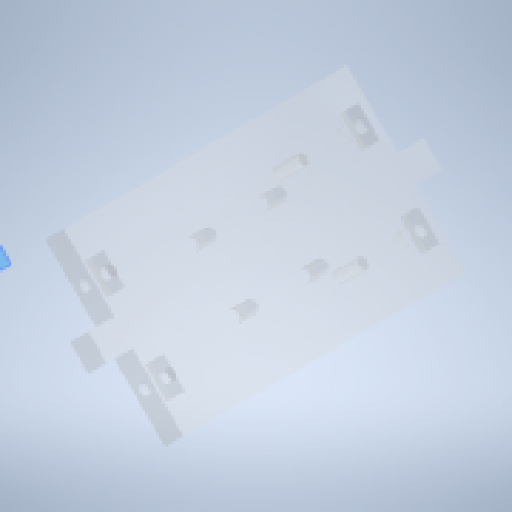
# Autodesk Inventor part: foot_2
Saved by Autodesk Inventor 2024 (Build 280153000, 153)
## iProperties
Created: 2024-09-05
Part Number: foot_2
Material: PMMA 플라스틱
Document SubType Name: Modeling
Designer: Eungang
Density: 1.188 g/cm^3
Appearance: 폴리카보네이트 - 선명
Mass: 18.11 g
Surface Area: 72.1845 cm^2
Volume: 15.2441 cm^3
Author: Eungang
Autodesk Inventor part; units mm, degrees
ref_plane "YZ Plane" through (0, 0, 0) normal (1, 0, 0) x (0, 1, 0)
ref_plane "XZ Plane" through (0, 0, 0) normal (0, 1, 0) x (-1, 0, 0)
ref_plane "XY Plane" through (0, 0, 0) normal (0, 0, 1) x (1, 0, 0)
sketch "스케치1" plane through (0, 0, 0) normal (0, 0, 1) x (1, 0, 0)
  arc A0 (25.8359, 13.6528) -> (21.7064, 16.0915) centre (22.8544, 13.3199) ccw projected
  line L0 (21.1279, 15.8519) -> (21.7064, 16.0915) projected
  arc A1 (21.1279, 15.8519) -> (19.2893, 12.7982) centre (22.276, 13.0803) ccw projected
  arc A2 (12.7982, 19.2893) -> (19.2893, 12.7982) centre (12.1212, 12.1212) ccw projected
  arc A3 (12.7982, 19.2893) -> (15.8519, 21.1279) centre (13.0803, 22.276) ccw projected
  line L1 (16.0915, 21.7064) -> (15.8519, 21.1279) projected
  arc A4 (16.0915, 21.7064) -> (13.6528, 25.8359) centre (13.3199, 22.8544) ccw projected
  arc A5 (13.6528, 25.8359) -> (2.3631, 21.8792) centre (12.1212, 12.1212) ccw projected
  line L2 (-25.9212, -6.405) -> (2.3631, 21.8792) projected
  line L3 (-18.2844, -14.0418) -> (-25.9212, -6.405) projected
  line L4 (-14.0418, -9.7991) -> (-18.2844, -14.0418) projected
  line L5 (-9.7991, -14.0418) -> (-14.0418, -9.7991) projected
  line L6 (-14.0418, -18.2844) -> (-9.7991, -14.0418) projected
  line L7 (-6.405, -25.9212) -> (-14.0418, -18.2844) projected
  line L8 (21.8792, 2.3631) -> (-6.405, -25.9212) projected
  arc A6 (21.8792, 2.3631) -> (25.8359, 13.6528) centre (12.1212, 12.1212) ccw projected
  circle A7 centre (23.1212, 12.1212) radius 1.2812 projected
  circle A8 centre (19.8993, 4.343) radius 1.2812 projected
  circle A9 centre (1.1212, 12.1212) radius 1.2812 projected
  circle A10 centre (12.1212, 1.1212) radius 1.2812 projected
  circle A11 centre (4.343, 4.343) radius 1.2812 projected
  circle A12 centre (4.343, 19.8993) radius 1.2812 projected
  circle A13 centre (12.1212, 23.1212) radius 1.2812 projected
  circle A14 centre (-7.1121, -20.9714) radius 1.25 projected
  circle A15 centre (-20.9714, -7.1121) radius 1.25 projected
  line L9 (-25.9212, -6.405) -> (-18.2844, -14.0418)
  line L10 (-14.0418, -9.7991) -> (-18.2844, -14.0418)
  line L11 (-14.0418, -9.7991) -> (-9.7991, -14.0418)
  line L12 (-14.0418, -18.2844) -> (-9.7991, -14.0418)
  line L13 (-21.6785, -2.1624) -> (-14.0418, -9.7991)
  line L14 (-21.6785, -2.1624) -> (-25.9212, -6.405)
  line L15 (-9.7991, -14.0418) -> (-2.1624, -21.6785)
  line L16 (-2.1624, -21.6785) -> (-6.405, -25.9212)
  line L17 (-6.405, -25.9212) -> (-14.0418, -18.2844)
  line L18 (-18.2844, -14.0418) -> (-14.0418, -18.2844)
  point P0 (0, 0)
  constraints: 20 end point, 6 collinear, 4 point on line, 2 perpendicular
extrude "돌출1" add sketch "스케치1" along normal blind 50.4 contours L8 L7 L6 L15 | L6 L18 L4 L5 | L4 L3 L2 L13 | A14 | A15
sketch "스케치2" plane through (0, 0, 0) normal (0, 0, -1) x (-1, 0, 0)
  line L0 (2.1624, -21.6785) -> (21.6785, -2.1624) projected
  arc A0 (-21.7064, 16.0915) -> (-25.8359, 13.6528) centre (-22.8544, 13.3199) ccw projected
  arc A1 (-25.8359, 13.6528) -> (-21.8792, 2.3631) centre (-12.1212, 12.1212) ccw projected
  line L1 (-21.8792, 2.3631) -> (6.405, -25.9212) projected
  line L2 (6.405, -25.9212) -> (14.0418, -18.2844) projected
  line L3 (14.0418, -18.2844) -> (9.7991, -14.0418) projected
  line L4 (9.7991, -14.0418) -> (14.0418, -9.7991) projected
  line L5 (14.0418, -9.7991) -> (18.2844, -14.0418) projected
  line L6 (18.2844, -14.0418) -> (25.9212, -6.405) projected
  line L7 (25.9212, -6.405) -> (-2.3631, 21.8792) projected
  arc A2 (-2.3631, 21.8792) -> (-13.6528, 25.8359) centre (-12.1212, 12.1212) ccw projected
  arc A3 (-13.6528, 25.8359) -> (-16.0915, 21.7064) centre (-13.3199, 22.8544) ccw projected
  line L8 (-16.0915, 21.7064) -> (-15.8519, 21.1279) projected
  arc A4 (-15.8519, 21.1279) -> (-12.7982, 19.2893) centre (-13.0803, 22.276) ccw projected
  arc A5 (-19.2893, 12.7982) -> (-12.7982, 19.2893) centre (-12.1212, 12.1212) ccw projected
  arc A6 (-19.2893, 12.7982) -> (-21.1279, 15.8519) centre (-22.276, 13.0803) ccw projected
  line L9 (-21.1279, 15.8519) -> (-21.7064, 16.0915) projected
  circle A7 centre (-23.1212, 12.1212) radius 1.2812 projected
  circle A8 centre (-19.8993, 4.343) radius 1.2812 projected
  circle A9 centre (-1.1212, 12.1212) radius 1.2812 projected
  circle A10 centre (-12.1212, 1.1212) radius 1.2812 projected
  circle A11 centre (-4.343, 4.343) radius 1.2812 projected
  circle A12 centre (-4.343, 19.8993) radius 1.2812 projected
  circle A13 centre (-12.1212, 23.1212) radius 1.2812 projected
  circle A14 centre (7.1121, -20.9714) radius 1.25 projected
  circle A15 centre (20.9714, -7.1121) radius 1.25 projected
  line L10 (25.9212, -6.405) -> (6.405, -25.9212) projected
  point P0 (0, 0)
extrude "돌출2" add sketch "스케치2" along normal blind 6 contours L0 L5 L10 L3
sketch "스케치3" plane through (0, 0, 50.4) normal (0, 0, 1) x (1, 0, 0)
  arc A0 (25.8359, 13.6528) -> (21.7064, 16.0915) centre (22.8544, 13.3199) ccw projected
  line L0 (21.1279, 15.8519) -> (21.7064, 16.0915) projected
  arc A1 (21.1279, 15.8519) -> (19.2893, 12.7982) centre (22.276, 13.0803) ccw projected
  arc A2 (12.7982, 19.2893) -> (19.2893, 12.7982) centre (12.1212, 12.1212) ccw projected
  arc A3 (12.7982, 19.2893) -> (15.8519, 21.1279) centre (13.0803, 22.276) ccw projected
  line L1 (16.0915, 21.7064) -> (15.8519, 21.1279) projected
  arc A4 (16.0915, 21.7064) -> (13.6528, 25.8359) centre (13.3199, 22.8544) ccw projected
  arc A5 (13.6528, 25.8359) -> (2.3631, 21.8792) centre (12.1212, 12.1212) ccw projected
  line L2 (-25.9212, -6.405) -> (2.3631, 21.8792) projected
  line L3 (-18.2844, -14.0418) -> (-25.9212, -6.405) projected
  line L4 (-14.0418, -9.7991) -> (-18.2844, -14.0418) projected
  line L5 (-9.7991, -14.0418) -> (-14.0418, -9.7991) projected
  line L6 (-14.0418, -18.2844) -> (-9.7991, -14.0418) projected
  line L7 (-6.405, -25.9212) -> (-14.0418, -18.2844) projected
  line L8 (21.8792, 2.3631) -> (-6.405, -25.9212) projected
  arc A6 (21.8792, 2.3631) -> (25.8359, 13.6528) centre (12.1212, 12.1212) ccw projected
  circle A7 centre (23.1212, 12.1212) radius 1.2812 projected
  circle A8 centre (19.8993, 4.343) radius 1.2812 projected
  circle A9 centre (1.1212, 12.1212) radius 1.2812 projected
  circle A10 centre (12.1212, 1.1212) radius 1.2812 projected
  circle A11 centre (4.343, 4.343) radius 1.2812 projected
  circle A12 centre (4.343, 19.8993) radius 1.2812 projected
  circle A13 centre (12.1212, 23.1212) radius 1.2812 projected
  circle A14 centre (-7.1121, -20.9714) radius 1.25 projected
  circle A15 centre (-20.9714, -7.1121) radius 1.25 projected
  line L9 (-25.9212, -6.405) -> (-6.405, -25.9212) projected
  point P0 (0, 0)
extrude "돌출3" add sketch "스케치3" along normal blind 6 contours L9 L4 L5 L6
sketch "스케치4" plane through (0, 0, 0) normal (0, 0, -1) x (-1, 0, 0)
  arc A0 (-21.7064, 16.0915) -> (-25.8359, 13.6528) centre (-22.8544, 13.3199) ccw projected
  arc A1 (-25.8359, 13.6528) -> (-21.8792, 2.3631) centre (-12.1212, 12.1212) ccw projected
  line L0 (-21.8792, 2.3631) -> (6.405, -25.9212) projected
  line L1 (6.405, -25.9212) -> (14.0418, -18.2844) projected
  line L2 (14.0418, -18.2844) -> (9.7991, -14.0418) projected
  line L3 (9.7991, -14.0418) -> (14.0418, -9.7991) projected
  line L4 (14.0418, -9.7991) -> (18.2844, -14.0418) projected
  line L5 (18.2844, -14.0418) -> (25.9212, -6.405) projected
  line L6 (25.9212, -6.405) -> (-2.3631, 21.8792) projected
  arc A2 (-2.3631, 21.8792) -> (-13.6528, 25.8359) centre (-12.1212, 12.1212) ccw projected
  arc A3 (-13.6528, 25.8359) -> (-16.0915, 21.7064) centre (-13.3199, 22.8544) ccw projected
  line L7 (-16.0915, 21.7064) -> (-15.8519, 21.1279) projected
  arc A4 (-15.8519, 21.1279) -> (-12.7982, 19.2893) centre (-13.0803, 22.276) ccw projected
  arc A5 (-19.2893, 12.7982) -> (-12.7982, 19.2893) centre (-12.1212, 12.1212) ccw projected
  arc A6 (-19.2893, 12.7982) -> (-21.1279, 15.8519) centre (-22.276, 13.0803) ccw projected
  line L8 (-21.1279, 15.8519) -> (-21.7064, 16.0915) projected
  circle A7 centre (-23.1212, 12.1212) radius 1.2812 projected
  circle A8 centre (-19.8993, 4.343) radius 1.2812 projected
  circle A9 centre (-1.1212, 12.1212) radius 1.2812 projected
  circle A10 centre (-12.1212, 1.1212) radius 1.2812 projected
  circle A11 centre (-4.343, 4.343) radius 1.2812 projected
  circle A12 centre (-4.343, 19.8993) radius 1.2812 projected
  circle A13 centre (-12.1212, 23.1212) radius 1.2812 projected
  circle A14 centre (7.1121, -20.9714) radius 1.25 projected
  circle A15 centre (20.9714, -7.1121) radius 1.25 projected
  point P0 (0, 0)
extrude "돌출4" cut sketch "스케치4" against normal blind 6 contours A14 | A15
sketch "스케치5" plane through (0, 0, 50.4) normal (0, 0, 1) x (1, 0, 0)
  arc A0 (25.8359, 13.6528) -> (21.7064, 16.0915) centre (22.8544, 13.3199) ccw projected
  line L0 (21.1279, 15.8519) -> (21.7064, 16.0915) projected
  arc A1 (21.1279, 15.8519) -> (19.2893, 12.7982) centre (22.276, 13.0803) ccw projected
  arc A2 (12.7982, 19.2893) -> (19.2893, 12.7982) centre (12.1212, 12.1212) ccw projected
  arc A3 (12.7982, 19.2893) -> (15.8519, 21.1279) centre (13.0803, 22.276) ccw projected
  line L1 (16.0915, 21.7064) -> (15.8519, 21.1279) projected
  arc A4 (16.0915, 21.7064) -> (13.6528, 25.8359) centre (13.3199, 22.8544) ccw projected
  arc A5 (13.6528, 25.8359) -> (2.3631, 21.8792) centre (12.1212, 12.1212) ccw projected
  line L2 (-25.9212, -6.405) -> (2.3631, 21.8792) projected
  line L3 (-18.2844, -14.0418) -> (-25.9212, -6.405) projected
  line L4 (-14.0418, -9.7991) -> (-18.2844, -14.0418) projected
  line L5 (-9.7991, -14.0418) -> (-14.0418, -9.7991) projected
  line L6 (-14.0418, -18.2844) -> (-9.7991, -14.0418) projected
  line L7 (-6.405, -25.9212) -> (-14.0418, -18.2844) projected
  line L8 (21.8792, 2.3631) -> (-6.405, -25.9212) projected
  arc A6 (21.8792, 2.3631) -> (25.8359, 13.6528) centre (12.1212, 12.1212) ccw projected
  circle A7 centre (23.1212, 12.1212) radius 1.2812 projected
  circle A8 centre (19.8993, 4.343) radius 1.2812 projected
  circle A9 centre (1.1212, 12.1212) radius 1.2812 projected
  circle A10 centre (12.1212, 1.1212) radius 1.2812 projected
  circle A11 centre (4.343, 4.343) radius 1.2812 projected
  circle A12 centre (4.343, 19.8993) radius 1.2812 projected
  circle A13 centre (12.1212, 23.1212) radius 1.2812 projected
  circle A14 centre (-7.1121, -20.9714) radius 1.25 projected
  circle A15 centre (-20.9714, -7.1121) radius 1.25 projected
  point P0 (0, 0)
extrude "돌출5" cut sketch "스케치5" against normal blind 6 contours A14 | A15
sketch "스케치16" plane through (-21.6785, -2.1624, 0) normal (0.7071068, 0.7071068, 0) x (-0.7071068, 0.7071068, 0)
  line L0 (-27.4, -20.9) -> (-27.4, -14.9) projected
  line L1 (-27.4, -14.9) -> (-17.8, -14.9) projected
  line L2 (-17.8, -14.9) -> (-17.8, -20.9) projected
  line L3 (-27.4, -20.9) -> (-17.8, -20.9) projected
  line L4 (0, 0) -> (0, 50.4) projected
  line L5 (-27.4, -14.9) -> (0, -14.9)
  line L6 (0, -14.9) -> (0, 0)
  line L7 (0, 0) -> (-27.4, 0)
  line L8 (-27.4, 0) -> (-27.4, -14.9)
  line L9 (-0.2, -14.9) -> (-0.2, -20.9) projected
  line L10 (-9.8, -20.9) -> (-0.2, -20.9) projected
  line L11 (-9.8, -20.9) -> (-9.8, -14.9) projected
  line L12 (-9.8, -14.9) -> (-0.2, -14.9) projected
  line L13 (-16.9, -20.9) -> (-16.9, -14.9) projected
  line L14 (-10.7, -20.9) -> (-10.7, -14.9) projected
  line L15 (-16.9, -14.9) -> (-10.7, -14.9)
  line L16 (-10.7, -14.9) -> (-10.7, -20.9)
  line L17 (-10.7, -20.9) -> (-16.9, -20.9)
  line L18 (-16.9, -20.9) -> (-16.9, -14.9)
  line L19 (-16.9, -14.9) -> (-16.8, -14.9)
  line L20 (-10.7, -14.9) -> (-10.8, -14.9)
  line L21 (-10.8, -14.9) -> (-10.8, -21)
  line L22 (-16.8, -14.9) -> (-16.8, -20.9)
  point P0 (-13.8, 0)
  point P1 (-16.8, -14.9)
  point P2 (-10.8, -20.9)
  dimension "d25" = 0.1
  dimension "d26" = 0.1
  constraints: 24 end point, 4 parallel, 4 perpendicular, 3 point on line, 2 horizontal
  measures "d25" distance of L13.end L19.end
  measures "d26" distance of L15.end L20.end
extrude "돌출11" add sketch "스케치16" against normal blind 6 contours L8 L7 L6 L5 L1 | L5 L21 L17 L22
sketch "스케치17" plane through (-14.0418, -9.7991, -14.9) normal (0, 0, -1) x (-0.7071068, -0.7071068, 0)
  line L0 (6, 10.6) -> (-34, 10.6) projected
  arc A0 (-34, 10.6) -> (-45.0739, 4.8949) centre (-34, -3) ccw projected
  arc A1 (-45.0739, 4.8949) -> (-43.6082, 2.05) centre (-43.6082, 3.85) ccw projected
  line L1 (-43.6082, 2.05) -> (-34, 2.05) projected
  arc A2 (-34, -8.05) -> (-34, 2.05) centre (-34, -3) ccw projected
  line L2 (-34, -8.05) -> (-43.6082, -8.05) projected
  arc A3 (-43.6082, -8.05) -> (-45.0739, -10.8949) centre (-43.6082, -9.85) ccw projected
  arc A4 (-45.0739, -10.8949) -> (-34, -16.6) centre (-34, -3) ccw projected
  line L3 (-34, -16.6) -> (6, -16.6) projected
  line L4 (6, -16.6) -> (6, -7) projected
  arc A5 (5.005, -6.1) -> (6, -7) centre (6, -6) ccw projected
  line L5 (5.005, -6.1) -> (0.995, -6.1) projected
  arc A6 (-0.1, -5.005) -> (0.995, -6.1) centre (0, -6) ccw projected
  line L6 (-0.1, -5.005) -> (-0.1, -0.995) projected
  arc A7 (0.995, 0.1) -> (-0.1, -0.995) centre (0, 0) ccw projected
  line L7 (0.995, 0.1) -> (5.005, 0.1) projected
  arc A8 (6, 1) -> (5.005, 0.1) centre (6, 0) ccw projected
  line L8 (6, 1) -> (6, 10.6) projected
  circle A9 centre (-34, -14) radius 1.2812 projected
  circle A10 centre (-41.7782, -10.7782) radius 1.2812 projected
  circle A11 centre (-23, -3) radius 1.2812 projected
  circle A12 centre (-26.2218, 4.7782) radius 1.2812 projected
  circle A13 centre (-26.2218, -10.7782) radius 1.2812 projected
  circle A14 centre (-34, 8) radius 1.2812 projected
  circle A15 centre (-41.7782, 4.7782) radius 1.2812 projected
  circle A16 centre (3, 6.8) radius 1.35
  circle A17 centre (3, -12.8) radius 1.35
  point P0 (-16.8581, -3)
  constraints: 2 centre point
extrude "돌출12" cut sketch "스케치17" against normal blind 6 contours A16 | A17
sketch "스케치18" plane through (0, 0, 50.4) normal (0, 0, 1) x (1, 0, 0)
  line L0 (2.5045, 21.7378) -> (-25.7798, -6.5464) projected
  line L1 (-18.9915, -13.3347) -> (-25.7798, -6.5464) projected
  arc A0 (-17.6516, -13.2675) -> (-18.9915, -13.3347) centre (-18.2844, -14.0418) ccw projected
  line L2 (-17.6516, -13.2675) -> (-14.8161, -10.432) projected
  arc A1 (-13.2675, -10.432) -> (-14.8161, -10.432) centre (-14.0418, -9.7991) ccw projected
  line L3 (-13.2675, -10.432) -> (-10.432, -13.2675) projected
  arc A2 (-10.432, -14.8161) -> (-10.432, -13.2675) centre (-9.7991, -14.0418) ccw projected
  line L4 (-10.432, -14.8161) -> (-13.2675, -17.6516) projected
  arc A3 (-13.3347, -18.9915) -> (-13.2675, -17.6516) centre (-14.0418, -18.2844) ccw projected
  line L5 (-6.5464, -25.7798) -> (-13.3347, -18.9915) projected
  line L6 (-6.5464, -25.7798) -> (21.7378, 2.5045) projected
  arc A4 (21.7378, 2.5045) -> (25.5341, 14.369) centre (12.1212, 12.1212) ccw projected
  arc A5 (25.5341, 14.369) -> (22.4861, 15.3443) centre (23.7589, 14.0715) ccw projected
  line L7 (22.4861, 15.3443) -> (15.6921, 8.5503) projected
  arc A6 (8.5503, 15.6921) -> (15.6921, 8.5503) centre (12.1212, 12.1212) ccw projected
  line L8 (8.5503, 15.6921) -> (15.3443, 22.4861) projected
  arc A7 (15.3443, 22.4861) -> (14.369, 25.5341) centre (14.0715, 23.7589) ccw projected
  arc A8 (14.369, 25.5341) -> (2.5045, 21.7378) centre (12.1212, 12.1212) ccw projected
  circle A9 centre (-7.1121, -20.9714) radius 1.25 projected
  circle A10 centre (12.1212, 23.1212) radius 1.2812 projected
  circle A11 centre (4.343, 19.8993) radius 1.2812 projected
  circle A12 centre (12.1212, 1.1212) radius 1.2812 projected
  circle A13 centre (1.1212, 12.1212) radius 1.2812 projected
  circle A14 centre (4.343, 4.343) radius 1.2812 projected
  circle A15 centre (23.1212, 12.1212) radius 1.2812 projected
  circle A16 centre (19.8993, 4.343) radius 1.2812 projected
  circle A17 centre (-20.9714, -7.1121) radius 1.25 projected
  circle A18 centre (-20.9714, -7.1121) radius 1.25 projected
  line L9 (-18.2844, -14.0418) -> (-14.0418, -9.7991) projected
  line L10 (-14.0418, -9.7991) -> (-21.6785, -2.1624) projected
  line L11 (-21.6785, -2.1624) -> (-25.9212, -6.405) projected
  line L12 (-25.9212, -6.405) -> (-18.2844, -14.0418) projected
  circle A19 centre (-7.1121, -20.9714) radius 1.25 projected
  line L13 (-9.7991, -14.0418) -> (-14.0418, -18.2844) projected
  line L14 (-14.0418, -18.2844) -> (-6.405, -25.9212) projected
  line L15 (-6.405, -25.9212) -> (-2.1624, -21.6785) projected
  line L16 (-2.1624, -21.6785) -> (-9.7991, -14.0418) projected
  point P0 (0, 0)
  point P1 (-21.5371, -2.3038)
  point P2 (-2.3038, -21.5371)
extrude "돌출13" cut sketch "스케치18" against normal through all contours L0 L12 L11 L10 | L16 L15 L14 L6
sketch "스케치20" plane through (-14.0418, -9.7991, 50.4) normal (0.7071068, 0.7071068, 0) x (-0.7071068, 0.7071068, 0)
  line L0 (10.6, -65.3) -> (10.6, 0) projected
  line L1 (0, 0) -> (10.6, 0) projected
  line L2 (0, 0) -> (0, 6) projected
  line L3 (-6, 6) -> (0, 6) projected
  line L4 (-6, 0) -> (-6, 6) projected
  line L5 (-16.6, 0) -> (-6, 0) projected
  line L6 (-16.6, 0) -> (-16.6, -65.3) projected
  line L7 (-16.6, -65.3) -> (-6, -65.3) projected
  line L8 (-6, -65.3) -> (-6, -71.3) projected
  line L9 (-6, -71.3) -> (0, -71.3) projected
  line L10 (0, -71.3) -> (0, -65.3) projected
  line L11 (0, -65.3) -> (10.6, -65.3) projected
  line L12 (-16.6, 0) -> (-16.6, -65.3) projected
  line L13 (-16.6, -32.65) -> (10.6, -32.65)
  line L14 (-3, 6) -> (-3, -71.3)
  line L15 (-3, -32.65) -> (-3, 0)
  line L16 (-5.005, 0) -> (-0.995, 0) projected
  line L17 (-3, 0) -> (-3, -32.65)
  line L18 (-6, -65.3) -> (0, -65.3)
  line L19 (-3, -65.3) -> (-3, -32.65)
  line L20 (-3, -48.975) -> (-16.6, -48.975)
  line L21 (-16.6, -65.3) -> (-16.6, 0) projected
  line L22 (-3, -48.975) -> (-3, -32.65)
  line L23 (-3, -40.8125) -> (-16.6, -40.8125)
  circle A0 centre (-9.8, -40.8125) radius 1.35
  circle A1 centre (3.8, -40.8125) radius 1.35
  circle A2 centre (-9.8, -24.4875) radius 1.35
  circle A3 centre (3.8, -24.4875) radius 1.35
  point P0 (-3, -50.4)
  dimension "d33" = 2.7
  constraints: 18 end point, 9 midpoint, 4 centre point, 4 perpendicular, 3 point on line, 3 symmetric about line, 2 collinear, 3 other
  measures "d33" diameter of A0
extrude "돌출14" cut sketch "스케치20" against normal up to next contours A0 L23 | L23 A0 | A1 | A2 | A3
sketch "스케치21" plane through (-14.0418, -9.7991, 50.4) normal (0.7071068, 0.7071068, 0) x (-0.7071068, 0.7071068, 0)
  circle A0 centre (3.8, -24.4875) radius 1.35 projected
  circle A1 centre (-9.8, -24.4875) radius 1.35 projected
  circle A2 centre (3.8, -40.8125) radius 1.35 projected
  circle A3 centre (-9.8, -40.8125) radius 1.35 projected
  line L0 (10.6, -65.3) -> (10.6, 0) projected
  line L1 (0, 0) -> (10.6, 0) projected
  line L2 (0, 0) -> (0, 6) projected
  line L3 (-6, 6) -> (0, 6) projected
  line L4 (-6, 0) -> (-6, 6) projected
  line L5 (-16.6, 0) -> (-6, 0) projected
  line L6 (-16.6, 0) -> (-16.6, -65.3) projected
  line L7 (-16.6, -65.3) -> (-6, -65.3) projected
  line L8 (-6, -65.3) -> (-6, -71.3) projected
  line L9 (-6, -71.3) -> (0, -71.3) projected
  line L10 (0, -71.3) -> (0, -65.3) projected
  line L11 (0, -65.3) -> (10.6, -65.3) projected
  line L12 (-11.55, 0) -> (-11.55, 6)
  line L13 (-11.55, 0) -> (-11.55, 6)
  line L14 (-14.05, 0) -> (-14.05, 6)
  line L15 (-14.05, -6) -> (-11.55, -6) projected
  line L16 (-11.55, 0) -> (-14.05, 0)
  line L17 (-14.05, 0) -> (-14.05, -6)
  line L18 (-14.05, -6) -> (-11.55, -6)
  line L19 (-11.55, -6) -> (-11.55, 0)
  line L20 (-12.8, -6) -> (-12.8, 0)
  line L21 (-12.8, -3) -> (-9.3, -3)
  line L22 (-12.8, -3) -> (-16.3, -3)
  line L23 (-9.3, -3) -> (-9.3, -4.5)
  line L24 (-9.3, -3) -> (-9.3, -1.5)
  line L25 (-16.3, -3) -> (-16.3, -4.5)
  line L26 (-16.3, -3) -> (-16.3, -1.5)
  line L27 (-9.3, -1.5) -> (-16.3, -1.5)
  line L28 (-16.3, -1.5) -> (-16.3, -4.5)
  line L29 (-16.3, -4.5) -> (-9.3, -4.5)
  line L30 (-9.3, -4.5) -> (-9.3, -1.5)
  line L31 (-3, 6) -> (-3, 1)
  line L32 (6.8, -3) -> (3.3, -3)
  line L33 (6.8, -3) -> (10.3, -3)
  line L34 (3.3, -3) -> (3.3, -4.5)
  line L35 (3.3, -3) -> (3.3, -1.5)
  line L36 (10.3, -3) -> (10.3, -4.5)
  line L37 (10.3, -3) -> (10.3, -1.5)
  line L38 (3.3, -1.5) -> (10.3, -1.5)
  line L39 (10.3, -1.5) -> (10.3, -4.5)
  line L40 (10.3, -4.5) -> (3.3, -4.5)
  line L41 (3.3, -4.5) -> (3.3, -1.5)
  line L42 (10.6, -32.65) -> (-16.6, -32.65)
  line L43 (-14.05, -59.3) -> (-11.55, -59.3)
  line L44 (-14.05, -59.3) -> (-11.55, -59.3)
  line L45 (-12.8, -62.3) -> (-9.3, -62.3)
  line L46 (-12.8, -62.3) -> (-16.3, -62.3)
  line L47 (-9.3, -62.3) -> (-9.3, -60.8)
  line L48 (-9.3, -62.3) -> (-9.3, -63.8)
  line L49 (-16.3, -62.3) -> (-16.3, -60.8)
  line L50 (-16.3, -62.3) -> (-16.3, -63.8)
  line L51 (-9.3, -63.8) -> (-16.3, -63.8)
  line L52 (-16.3, -63.8) -> (-16.3, -60.8)
  line L53 (-16.3, -60.8) -> (-9.3, -60.8)
  line L54 (-9.3, -60.8) -> (-9.3, -63.8)
  line L55 (10.3, -60.8) -> (3.3, -60.8)
  line L56 (10.3, -62.3) -> (10.3, -60.8)
  line L57 (3.3, -62.3) -> (3.3, -60.8)
  line L58 (6.8, -62.3) -> (3.3, -62.3)
  line L59 (6.8, -62.3) -> (10.3, -62.3)
  line L60 (3.3, -62.3) -> (3.3, -63.8)
  line L61 (3.3, -60.8) -> (3.3, -63.8)
  line L62 (3.3, -63.8) -> (10.3, -63.8)
  line L63 (10.3, -62.3) -> (10.3, -63.8)
  line L64 (10.3, -63.8) -> (10.3, -60.8)
  line L65 (10.6, 0) -> (16.6, 0)
  line L66 (16.6, 0) -> (16.6, -65.3)
  line L67 (16.6, -65.3) -> (10.6, -65.3)
  line L68 (10.6, -65.3) -> (10.6, 0)
  line L69 (-16.6, 0) -> (-22.6, 0)
  line L70 (-22.6, 0) -> (-22.6, -65.3)
  line L71 (-22.6, -65.3) -> (-16.6, -65.3)
  line L72 (-16.6, -65.3) -> (-16.6, 0)
  point P0 (-3, -50.4)
  point P1 (-16.3, -1.5)
  point P2 (-9.3, -4.5)
  point P3 (3.3, -4.5)
  point P4 (10.3, -1.5)
  point P5 (-12.8, -59.3)
  dimension "d36" = 3.5
  dimension "d37" = 3.5
  dimension "d38" = 1.5
  dimension "d39" = 1.5
  dimension "d40" = 1.5
  dimension "d43" = 6
  dimension "d44" = 6
  constraints: 120 end point, 31 symmetric about line, 8 parallel, 8 vertical, 6 midpoint, 5 perpendicular, 5 point on line, 4 horizontal, 4 other
  measures "d36" distance of L21.start L21.end
  measures "d37" distance of L21.start L22.end
  measures "d38" distance of L21.end L23.end
  measures "d39" distance of L21.end L24.end
  measures "d40" distance of L22.end L25.end
  measures "d43" distance of L66.end L67.end
  measures "d44" distance of L71.end L70.end
extrude "돌출15" cut sketch "스케치21" against normal up to next contours L27 L20 L22 L17 | L17 L22 L26 L27 | L27 L19 L21 L20 | L22 L20 L29 L17 | L17 L29 L25 L22 | L27 L24 L21 L19 | L21 L19 L29 L20 | L21 L23 L29 L19 | L33 L36 L40 L34 L32 | L32 L35 L38 L37 L33
sketch "스케치22" plane through (-14.0418, -9.7991, 50.4) normal (0.7071068, 0.7071068, 0) x (-0.7071068, 0.7071068, 0)
  line L0 (-9.3, -4.5) -> (-16.3, -4.5) projected
  line L1 (-16.3, -4.5) -> (-16.3, -1.5) projected
  line L2 (-16.3, -1.5) -> (-9.3, -1.5) projected
  line L3 (-9.3, -1.5) -> (-9.3, -4.5) projected
  line L4 (3.3, -1.5) -> (10.3, -1.5) projected
  line L5 (10.3, -1.5) -> (10.3, -4.5) projected
  line L6 (10.3, -4.5) -> (3.3, -4.5) projected
  line L7 (3.3, -4.5) -> (3.3, -1.5) projected
  circle A0 centre (3.8, -24.4875) radius 1.35 projected
  circle A1 centre (-9.8, -24.4875) radius 1.35 projected
  circle A2 centre (3.8, -40.8125) radius 1.35 projected
  circle A3 centre (-9.8, -40.8125) radius 1.35 projected
  line L8 (10.6, -65.3) -> (10.6, 0) projected
  line L9 (0, 0) -> (10.6, 0) projected
  line L10 (0, 0) -> (0, 6) projected
  line L11 (-6, 6) -> (0, 6) projected
  line L12 (-6, 0) -> (-6, 6) projected
  line L13 (-16.6, 0) -> (-6, 0) projected
  line L14 (-16.6, 0) -> (-16.6, -65.3) projected
  line L15 (-16.6, -65.3) -> (-6, -65.3) projected
  line L16 (-6, -65.3) -> (-6, -71.3) projected
  line L17 (-6, -71.3) -> (0, -71.3) projected
  line L18 (0, -71.3) -> (0, -65.3) projected
  line L19 (0, -65.3) -> (10.6, -65.3) projected
  line L20 (10.6, -65.3) -> (10.6, 0) projected
  line L21 (10.6, -32.65) -> (-17.5141, -32.65)
  line L22 (-9.3, -60.8) -> (-16.3, -60.8)
  line L23 (-16.3, -60.8) -> (-16.3, -63.8)
  line L24 (-16.3, -63.8) -> (-9.3, -63.8)
  line L25 (-9.3, -63.8) -> (-9.3, -60.8)
  line L26 (3.3, -63.8) -> (10.3, -63.8)
  line L27 (10.3, -63.8) -> (10.3, -60.8)
  line L28 (10.3, -60.8) -> (3.3, -60.8)
  line L29 (3.3, -60.8) -> (3.3, -63.8)
  line L30 (10.6, 0) -> (16.6, 0)
  line L31 (16.6, 0) -> (16.6, -65.3)
  line L32 (16.6, -65.3) -> (10.6, -65.3)
  line L33 (10.6, -65.3) -> (10.6, 0)
  line L34 (-16.6, 0) -> (-22.6, 0)
  line L35 (-22.6, 0) -> (-22.6, -65.3)
  line L36 (-22.6, -65.3) -> (-16.6, -65.3)
  line L37 (-16.6, -65.3) -> (-16.6, 0)
  point P0 (-3, -50.4)
  point P1 (10.6, -65.3)
  dimension "d45" = 6
  dimension "d46" = 6
  constraints: 34 end point, 8 symmetric about line, 4 parallel, 3 horizontal, 2 perpendicular, 1 midpoint, 1 point on line
  measures "d45" distance of L31.end L32.end
  measures "d46" distance of L36.end L35.end
extrude "돌출16" add sketch "스케치22" against normal blind 6 contours L8 L30 L31 L32 | L14 L36 L35 L34
thicken "두껍게 하기1" operation add thickness 0.19 both sides no extend neighbours no toward (0, 0, 1) faces at (-25.9031, -2.2161, 50.4)
thicken "두껍게 하기2" operation add thickness 0.19 both sides no extend neighbours no toward (0, 0, 1) faces at (-2.1805, -25.8675, 50.4)
thicken "두껍게 하기3" operation add thickness 0.1 both sides no extend neighbours no toward (0, 0, 1) faces at (-25.9031, -2.2161, 50.59)
thicken "두껍게 하기4" operation add thickness 0.1 both sides no extend neighbours no toward (0, 0, 1) faces at (-2.1805, -25.8675, 50.59)
thicken "두껍게 하기5" operation add thickness 0.29 both sides no extend neighbours no toward (0, 0, 1) faces at (-12.6276, -14.0418, 56.4)
thicken "두껍게 하기6" operation add thickness 0.01 both sides no extend neighbours no toward (0, 0, 1) faces at (-25.9031, -2.2161, 50.69)
thicken "두껍게 하기7" operation add thickness 0.01 both sides no extend neighbours no toward (0, 0, 1) faces at (-12.6276, -14.0418, 56.69)
thicken "두껍게 하기8" operation add thickness 0.01 both sides no extend neighbours no toward (0, 0, 1) faces at (-2.1805, -25.8675, 50.69)
sketch "스케치23" plane through (-9.7991, -14.0418, -20.9) normal (0.7071068, 0.7071068, 0) x (-0.7071068, 0.7071068, 0)
  line L0 (-3.3, 66.8) -> (-10.3, 66.8) projected
  line L1 (-10.3, 66.8) -> (-10.3, 69.8) projected
  line L2 (-10.3, 69.8) -> (-3.3, 69.8) projected
  line L3 (-3.3, 69.8) -> (-3.3, 66.8) projected
  line L4 (9.3, 69.8) -> (16.3, 69.8) projected
  line L5 (16.3, 69.8) -> (16.3, 66.8) projected
  line L6 (16.3, 66.8) -> (9.3, 66.8) projected
  line L7 (9.3, 66.8) -> (9.3, 69.8) projected
  circle A0 centre (9.8, 46.8125) radius 1.35 projected
  circle A1 centre (-3.8, 46.8125) radius 1.35 projected
  circle A2 centre (9.8, 30.4875) radius 1.35 projected
  circle A3 centre (-3.8, 30.4875) radius 1.35 projected
  line L8 (6, 71.6) -> (6, 77.6) projected
  line L9 (0, 77.6) -> (6, 77.6) projected
  line L10 (0, 71.6) -> (0, 77.6) projected
  line L11 (-16.6, 71.6) -> (0, 71.6) projected
  line L12 (-16.6, 71.6) -> (-16.6, 6) projected
  line L13 (-16.6, 6) -> (0, 6) projected
  line L14 (0, 6) -> (0, 0) projected
  line L15 (0, 0) -> (6, 0) projected
  line L16 (6, 0) -> (6, 6) projected
  line L17 (6, 6) -> (22.6, 6) projected
  line L18 (22.6, 6) -> (22.6, 71.6) projected
  line L19 (6, 71.6) -> (22.6, 71.6) projected
  circle A4 centre (-3.8, 46.8125) radius 1.35 projected
  line L20 (-3.8, 46.8125) -> (-3.8, 30.4875)
  line L21 (-16.6, 71.6) -> (-16.6, 6) projected
  line L22 (-16.6, 38.8) -> (22.6, 38.8)
  line L23 (-3.3, 10.8) -> (-10.3, 10.8)
  line L24 (-10.3, 10.8) -> (-10.3, 7.8)
  line L25 (-10.3, 7.8) -> (-3.3, 7.8)
  line L26 (-3.3, 7.8) -> (-3.3, 10.8)
  line L27 (9.3, 7.8) -> (16.3, 7.8)
  line L28 (16.3, 7.8) -> (16.3, 10.8)
  line L29 (16.3, 10.8) -> (9.3, 10.8)
  line L30 (9.3, 10.8) -> (9.3, 7.8)
  line L31 (-16.6, 6) -> (0, 6)
  point P0 (3, 20.9)
  constraints: 22 end point, 8 symmetric about line, 2 midpoint, 1 vertical
extrude "돌출17" cut sketch "스케치23" against normal up to next contours L26 L25 L24 L23 | L30 L29 L28 L27
